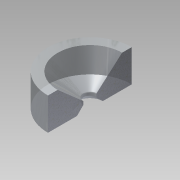
# Autodesk Inventor part: nozzle_big
Saved by Autodesk Inventor 2014 (Build 180170000, 170)
## iProperties
Created: 2013-10-01
Part Number: nozzle_big
Material: Glass
Document SubType Name: Modeling
Designer: Admin
Density: 1 g/cm^3
Appearance: Clear
Author: Admin
Autodesk Inventor part; units mm, degrees
ref_plane "YZ Plane" through (0, 0, 0) normal (1, 0, 0) x (0, 1, 0)
ref_plane "XZ Plane" through (0, 0, 0) normal (0, 1, 0) x (-1, 0, 0)
ref_plane "XY Plane" through (0, 0, 0) normal (0, 0, 1) x (1, 0, 0)
sketch "Sketch2" plane through (0, 0, 0) normal (0, 1, 0) x (-1, 0, 0)
  line L0 (6.5, 0) -> (6.5, 5)
  line L1 (6.5, 5) -> (5, 5)
  line L2 (6.5, 5) -> (6.5, 0)
  line L3 (0, -1) -> (0, 6) projected
  line L4 (6.5, 0) -> (2, 0)
  line L5 (2, 0) -> (1, 1)
  line L6 (1, 1) -> (1, 1.5)
  line L7 (5, 5) -> (1, 1.5)
  point P0 (0, 0)
  dimension "d4" = 5
  dimension "d5" = 1.5
  dimension "d11" = 6.5
  dimension "d26" = 4.5
  dimension "d27" = 0.5
  dimension "d28" = 1
  dimension "d29" = 2
  dimension "d31" = 1
  constraints: 14 end point, 3 perpendicular
  measures "d4" distance of L0.start L0.end
  measures "d5" distance of L0.end L1.end
  measures "d11" distance of L0.start point (0, 0)
  measures "d26" distance of L0.start L4.end
  measures "d27" distance of L5.end L6.end
  measures "d28" horizontal distance of point (0, 0) L5.end
  measures "d29" distance of point (0, 0) L4.end
  measures "d31" horizontal distance of point (0, 0) L5.end
revolve "Revolution2" add sketch "Sketch2" angle 360 about axis through (0, 0, -10) along (0, 0, 1)
fillet "Fillet4" radius 0.2 2 edges at (1, 0, 1) (1, 0, 1.5)
body "Solid2"
